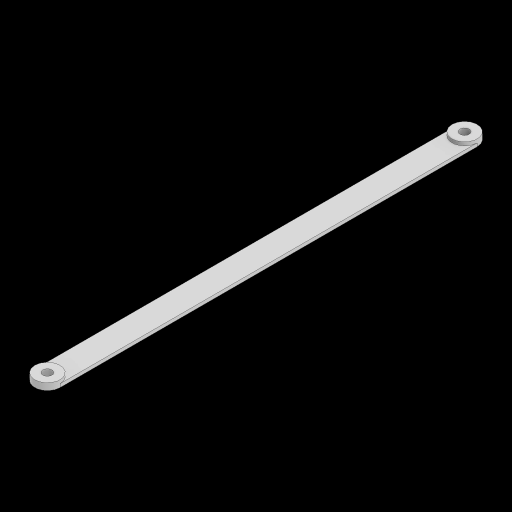
# Autodesk Inventor part: közepső szalag 1
Saved by Autodesk Inventor 2023 (Build 270158000, 158)
## iProperties
Created: 2022-11-11
Part Number: közepső szalag 1
Material: Generic
Document SubType Name: Modeling
Designer: gd1
Density: 1 g/cm^3
Appearance: Default
Author: gd1
Autodesk Inventor part; units mm, degrees
ref_plane "YZ Plane" through (0, 0, 0) normal (1, 0, 0) x (0, 1, 0)
ref_plane "XZ Plane" through (0, 0, 0) normal (0, 1, 0) x (-1, 0, 0)
ref_plane "XY Plane" through (0, 0, 0) normal (0, 0, 1) x (1, 0, 0)
sketch "Sketch1" plane through (0, 0, 0) normal (0, 1, 0) x (-1, 0, 0)
  circle A0 centre (0, 0) radius 7.5
  circle A1 centre (0, 0) radius 2.75
  line L0 (0, -255.47) -> (0, 0) construction
  line L1 (-7.5, -247.97) -> (-7.5, 0)
  line L2 (7.5, 0) -> (7.5, -247.97)
  arc A2 (7.5, 0) -> (-7.5, 0) centre (0, 0) ccw
  line L3 (0, -255.47) -> (0, -240.47)
  circle A3 centre (0, -247.97) radius 2.75
  circle A4 centre (0, -247.97) radius 7.5
  point P0 (0, -127.735)
  point P1 (7.5, 0)
  point P2 (-7.5, 0)
  point P3 (0, 7.5)
  dimension "d0" = 15
  dimension "d1" = 5.5
  dimension "d7" = 15
  dimension "d12" = 15
  dimension "d13" = 5.5
  dimension "d17" = 262.97
  constraints: 9 end point, 6 point on circle, 5 centre point, 3 coincident, 2 midpoint, 2 tangent, 1 parallel, 1 point on line, 1 vertical
  measures "d0" diameter of A0
  measures "d1" diameter of A1
  measures "d7" distance between parallel lines of L1 L2
  measures "d12" distance of L0.start L3.end
  measures "d13" diameter of A3
  measures "d17" distance of point (0, 7.5) L0.start
extrude "Extrusion2" add sketch "Sketch1" along normal blind 4 contours A0 | A4 L3 A3 | A4 L3 A3
extrude "Extrusion3" add sketch "Sketch1" along normal blind 2 contours L2 A4 L1 A0
body "Solid1"
